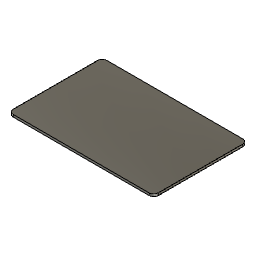
NamePlate (Autodesk Fusion 360 design; units mm, degrees)
Autodesk Fusion 360 part; units mm, degrees
note: some values were not read from the file. Set by a fixed rule: which sketch regions a step uses.
sketch "Sketch1" plane through (0, 0, 0) normal (0, 0, 1) x (1, 0, 0)
  line L0 (1.524, 0) -> (46.482, 0)
  line L1 (48.006, 1.524) -> (48.006, 29.464)
  line L2 (46.482, 30.988) -> (1.524, 30.988)
  line L3 (0, 29.464) -> (0, 1.524)
  arc A0 (1.524, 30.988) -> (0, 29.464) centre (1.524, 29.464) ccw
  arc A1 (0, 1.524) -> (1.524, 0) centre (1.524, 1.524) ccw
  arc A2 (48.006, 29.464) -> (46.482, 30.988) centre (46.482, 29.464) ccw
  arc A3 (46.482, 0) -> (48.006, 1.524) centre (46.482, 1.524) ccw
  point P0 (48.006, 0)
  point P1 (0, 30.988)
  dimension "d1" = 48.006
  dimension "d2" = 30.988
  dimension "d5" = 1.524
  dimension "d6" = 1.524
  dimension "d7" = 1.524
  dimension "d8" = 1.524
  constraint horizontal L0
  constraint vertical L1
  constraint horizontal L2
  constraint vertical L3
  constraint coincident P1 L2
  constraint coincident P1 L3
  constraint tangent L2 A0
  constraint tangent L3 A0
  constraint coincident origin L0
  constraint coincident origin L3
  constraint tangent L0 A1
  constraint tangent L3 A1
  constraint tangent L1 A2
  constraint tangent L2 A2
  constraint coincident P0 L0
  constraint coincident P0 L1
  constraint tangent L0 A3
  constraint tangent L1 A3
  measures "d1" distance of origin P0
  measures "d2" distance of origin P1
  measures "d5" radius of A0
  measures "d6" radius of A1
  measures "d7" radius of A2
  measures "d8" radius of A3
extrude "Extrude1" add sketch "Sketch1" along normal blind 0.762
